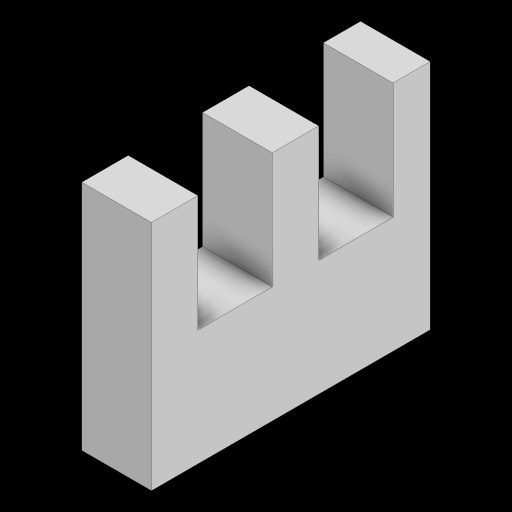
# Autodesk Inventor part: Sostenedor_inf
Saved by Autodesk Inventor 2024.2 (Build 282272000, 272)
## iProperties
Created: 2024-10-01
Part Number: Sostenedor_inf
Material: Generic
Document SubType Name: Modeling
Designer: jrcer
Density: 1 g/cm^3
Appearance: Default
Author: jrcer
Autodesk Inventor part; units mm, degrees
ref_plane "YZ Plane" through (0, 0, 0) normal (1, 0, 0) x (0, 1, 0)
ref_plane "XZ Plane" through (0, 0, 0) normal (0, 1, 0) x (-1, 0, 0)
ref_plane "XY Plane" through (0, 0, 0) normal (0, 0, 1) x (1, 0, 0)
sketch "Sketch1" plane through (0, 0, 0) normal (1, 0, 0) x (0, 1, 0)
  line L0 (0, 0) -> (10, 0)
  line L1 (10, 0) -> (10, -12)
  line L2 (10, -12) -> (0, -12)
  line L3 (0, -12) -> (0, 0)
  line L4 (10, -2) -> (5, -2)
  line L5 (5, -2) -> (5, -5.2)
  line L6 (5, -5.2) -> (10, -5.2)
  line L7 (10, -5.2) -> (10, -2)
  line L8 (10, -7.2) -> (5, -7.2)
  line L9 (5, -7.2) -> (5, -10.4)
  line L10 (5, -10.4) -> (10, -10.4)
  line L11 (10, -10.4) -> (10, -7.2)
  point P0 (5, 0)
  point P1 (10, -5.2)
  dimension "d0" = 10
  dimension "d1" = 12
  dimension "d2" = 5
  dimension "d3" = 3.2
  dimension "d4" = 2
  dimension "d5" = 2
  constraints: 24 end point, 6 parallel, 3 horizontal, 3 perpendicular, 3 point on line, 1 collinear, 1 midpoint
  measures "d0" distance of L1.end L2.end
  measures "d1" distance of L0.end L1.end
  measures "d2" distance of L6.end L5.end
  measures "d3" distance of L5.end L4.end
  measures "d4" distance from line of point (5, 0) L4
  measures "d5" distance between parallel lines of L8 L6
extrude "Extrusion1" add sketch "Sketch1" along normal blind 3 contours L0 L1 L4 L5 L6 L8 L9 L10 L2 L3
body "Solid1"
